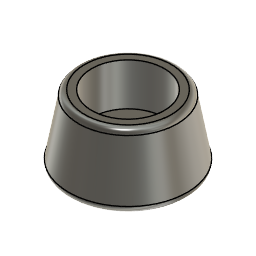
endcap-v1 (Autodesk Fusion 360 design; units mm, degrees)
part number: 2026-01-03-12-10-12-596
part number: 2026-01-03-12-10-40-974
Autodesk Fusion 360 part; units mm, degrees
sketch "Sketch1" plane through (0, 0, 0) normal (0, 0, 1) x (1, 0, 0) in component "Component"
  circle A0 centre (0, 0) radius 3
  circle A1 centre (0, 0) radius 4
  dimension "d1" = 6
  dimension "d2" = 8
  constraint coincident A0.centre A1.centre
  constraint concentric A0 A1
  measures "d1" diameter of A0
  measures "d2" diameter of A1
extrude "Extrude1" add sketch "Sketch1" along normal blind 3.5 in component "Component"
sketch "Sketch2" plane through (0, 0, 3.5) normal (0, 0, 1) x (-1, 0, 0) in component "Component"
  circle A0 centre (0, 0) radius 3
  circle A1 centre (0, 0) radius 4
  circle A2 centre (0, 0) radius 1.5
  dimension "d5" = 3
  measures "d5" diameter of A2
extrude "Extrude2" add sketch "Sketch2" along normal blind 2 contours A0 | A1 in component "Component"
sketch "Sketch3" plane through (0, 0, 5.5) normal (0, 0, 1) x (-1, 0, 0) in component "Component"
  circle A0 centre (0, 0) radius 1.5
  circle A1 centre (0, 0) radius 4
sketch "Sketch4" plane through (0, 0, 5.5) normal (0, 0, 1) x (1, 0, 0) in component "Component"
  circle A0 centre (0, 0) radius 5
  dimension "d8" = 10
  constraint coincident A0.centre origin
  measures "d8" diameter of A0
sketch "Sketch5" plane through (0, 0, 5.5) normal (0, 0, 1) x (1, 0, 0) in component "Component"
sketch "Sketch6" plane through (0, 0, 0) normal (0, 1, 0) x (1, 0, 0) in component "Component"
  line L0 (4, 0) -> (5, -5.5)
  line L1 (4, 0) -> (4, -5.5)
  line L2 (4, -5.5) -> (5, -5.5)
  constraint vertical L1
sketch "Sketch7" plane through (0, 0, 5.5) normal (0, 0, 1) x (1, 0, 0) in component "Component"
sketch "Sketch8" plane through (0, 0, 0) normal (0, 1, 0) x (1, 0, 0) in component "Component"
  line L0 (0, -5.5) -> (0, 0)
  constraint coincident L0.end origin
  constraint vertical L0
revolve "Revolve1" add sketch "Sketch6" angle 360 about axis through (0, 0, 5.5) along (0, 0, -1) in component "Component"
fillet "Fillet1" radius 0.5 1 edges at (-4.6616, -1.8081, 5.5) in component "Component"
fillet "Fillet2" radius 0.5 1 edges at (-3.7293, -1.4465, 0) in component "Component"
sketch "Sketch9" plane through (0, 0, 0) normal (0, 1, 0) x (1, 0, 0) in component "Component"
sketch "Sketch10" plane through (0, 0, 0) normal (0, 1, 0) x (1, 0, 0) in component "Component"
  line L0 (4, -2.75) -> (1, -2.75)
component "Component" placed x (1, 0, 0) y (0, 1, 0) z (0, 0, 1) at (0, 0, 0)
